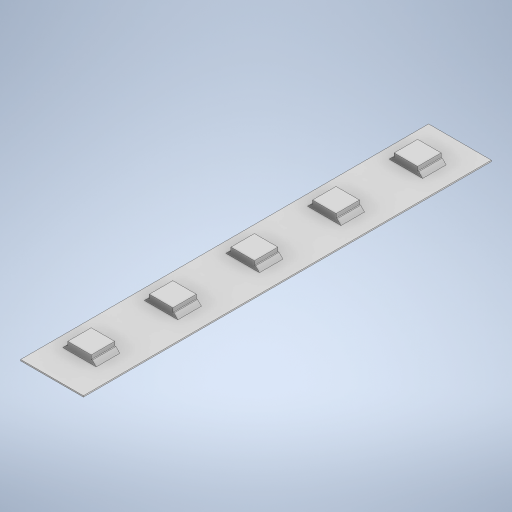
# Autodesk Inventor part: LED_Strip
Saved by Autodesk Inventor 2023 (Build 270158000, 158)
## iProperties
Created: 2022-12-07
Part Number: LED_Strip
Material: Generic
Document SubType Name: Modeling
Designer: spfow
Density: 1 g/cm^3
Appearance: Default
Author: spfow
Autodesk Inventor part; units mm, degrees
ref_plane "YZ Plane" through (0, 0, 0) normal (1, 0, 0) x (0, 1, 0)
ref_plane "XZ Plane" through (0, 0, 0) normal (0, 1, 0) x (-1, 0, 0)
ref_plane "XY Plane" through (0, 0, 0) normal (0, 0, 1) x (1, 0, 0)
sketch "Sketch1" plane through (0, 0, 0) normal (0, 1, 0) x (-1, 0, 0)
  line L0 (0, 0) -> (12.7, 0)
  line L1 (12.7, 0) -> (12.7, 82.55)
  line L2 (12.7, 82.55) -> (0, 82.55)
  line L3 (0, 82.55) -> (0, 0)
  dimension "d0" = 12.7
  dimension "d1" = 82.55
  constraints: 8 end point, 2 parallel, 1 horizontal, 1 perpendicular
  measures "d0" distance of L2.end L1.end
  measures "d1" distance of L0.end L1.end
extrude "Extrusion1" add sketch "Sketch1" along normal blind 0.254
sketch "Sketch2" plane through (0, 0.254, 0) normal (0, 1, 0) x (1, 0, 0)
  line L0 (-9.525, -76.2) -> (-4.7625, -76.2)
  line L1 (-4.7625, -76.2) -> (-4.7625, -71.4375)
  line L2 (-4.7625, -71.4375) -> (-9.525, -71.4375)
  line L3 (-9.525, -71.4375) -> (-9.525, -76.2)
  line L4 (-12.7, -82.55) -> (0, -82.55) projected
  line L5 (-12.7, 0) -> (-12.7, -82.55) projected
  line L6 (-9.525, -59.69) -> (-4.7625, -59.69)
  line L7 (-4.7625, -59.69) -> (-4.7625, -54.9275)
  line L8 (-4.7625, -54.9275) -> (-9.525, -54.9275)
  line L9 (-9.525, -54.9275) -> (-9.525, -59.69)
  line L10 (-9.525, -43.18) -> (-4.7625, -43.18)
  line L11 (-4.7625, -43.18) -> (-4.7625, -38.4175)
  line L12 (-4.7625, -38.4175) -> (-9.525, -38.4175)
  line L13 (-9.525, -38.4175) -> (-9.525, -43.18)
  line L14 (-9.525, -26.67) -> (-4.7625, -26.67)
  line L15 (-4.7625, -26.67) -> (-4.7625, -21.9075)
  line L16 (-4.7625, -21.9075) -> (-9.525, -21.9075)
  line L17 (-9.525, -21.9075) -> (-9.525, -26.67)
  line L18 (-9.525, -10.16) -> (-4.7625, -10.16)
  line L19 (-4.7625, -10.16) -> (-4.7625, -5.3975)
  line L20 (-4.7625, -5.3975) -> (-9.525, -5.3975)
  line L21 (-9.525, -5.3975) -> (-9.525, -10.16)
  line L22 (-4.7625, -59.69) -> (-3.7465, -59.69)
  line L23 (-3.7465, -59.69) -> (-3.7465, -54.9275)
  line L24 (-3.7465, -54.9275) -> (-4.7625, -54.9275)
  line L25 (-4.7625, -54.9275) -> (-4.7625, -59.69)
  line L26 (-4.7625, -76.2) -> (-3.7465, -76.2)
  line L27 (-3.7465, -76.2) -> (-3.7465, -71.4375)
  line L28 (-3.7465, -71.4375) -> (-4.7625, -71.4375)
  line L29 (-4.7625, -71.4375) -> (-4.7625, -76.2)
  line L30 (-9.525, -76.2) -> (-10.541, -76.2)
  line L31 (-10.541, -76.2) -> (-10.541, -71.4375)
  line L32 (-10.541, -71.4375) -> (-9.525, -71.4375)
  line L33 (-9.525, -71.4375) -> (-9.525, -76.2)
  line L34 (-9.525, -59.69) -> (-10.541, -59.69)
  line L35 (-10.541, -59.69) -> (-10.541, -54.9275)
  line L36 (-10.541, -54.9275) -> (-9.525, -54.9275)
  line L37 (-9.525, -54.9275) -> (-9.525, -59.69)
  line L38 (-9.525, -43.18) -> (-10.541, -43.18)
  line L39 (-10.541, -43.18) -> (-10.541, -38.4175)
  line L40 (-10.541, -38.4175) -> (-9.525, -38.4175)
  line L41 (-9.525, -38.4175) -> (-9.525, -43.18)
  line L42 (-4.7625, -43.18) -> (-3.7465, -43.18)
  line L43 (-3.7465, -43.18) -> (-3.7465, -38.4175)
  line L44 (-3.7465, -38.4175) -> (-4.7625, -38.4175)
  line L45 (-4.7625, -38.4175) -> (-4.7625, -43.18)
  line L46 (-4.7625, -26.67) -> (-3.7465, -26.67)
  line L47 (-3.7465, -26.67) -> (-3.7465, -21.9075)
  line L48 (-3.7465, -21.9075) -> (-4.7625, -21.9075)
  line L49 (-4.7625, -21.9075) -> (-4.7625, -26.67)
  line L50 (-9.525, -26.67) -> (-10.541, -26.67)
  line L51 (-10.541, -26.67) -> (-10.541, -21.9075)
  line L52 (-10.541, -21.9075) -> (-9.525, -21.9075)
  line L53 (-9.525, -21.9075) -> (-9.525, -26.67)
  line L54 (-9.525, -10.16) -> (-10.541, -10.16)
  line L55 (-10.541, -10.16) -> (-10.541, -5.3975)
  line L56 (-10.541, -5.3975) -> (-9.525, -5.3975)
  line L57 (-9.525, -5.3975) -> (-9.525, -10.16)
  line L58 (-4.7625, -10.16) -> (-3.7465, -10.16)
  line L59 (-3.7465, -10.16) -> (-3.7465, -5.3975)
  line L60 (-3.7465, -5.3975) -> (-4.7625, -5.3975)
  line L61 (-4.7625, -5.3975) -> (-4.7625, -10.16)
  point P0 (0, 0)
  point P1 (-4.7625, -21.9075)
  point P2 (-4.7625, -54.9275)
  dimension "d4" = 4.7625
  dimension "d5" = 4.7625
  dimension "d6" = 6.35
  dimension "d7" = 3.175
  dimension "d8" = 4.7625
  dimension "d9" = 4.7625
  dimension "d10" = 11.7475
  dimension "d11" = 3.175
  dimension "d12" = 4.7625
  dimension "d13" = 4.7625
  dimension "d14" = 4.7625
  dimension "d15" = 4.7625
  dimension "d16" = 4.7625
  dimension "d17" = 4.7625
  dimension "d18" = 11.7475
  dimension "d19" = 11.7475
  dimension "d20" = 11.7475
  dimension "d21" = 3.175
  dimension "d22" = 1.016
  dimension "d23" = 1.016
  dimension "d31" = 4.7625
  dimension "d32" = 4.7625
  dimension "d33" = 4.7625
  dimension "d34" = 4.7625
  constraints: 120 end point, 30 parallel, 17 point on line, 15 horizontal, 15 perpendicular
  measures "d4" distance of L2.end L0.start
  measures "d5" distance of L0.start L0.end
  measures "d6" distance between parallel lines of L4 L0
  measures "d7" distance between parallel lines of L5 L3
  measures "d8" distance of L8.end L6.start
  measures "d9" distance of L7.end L8.end
  measures "d10" distance between parallel lines of L6 L2
  measures "d11" distance between parallel lines of L5 L9
  measures "d12" distance of L11.end L12.end
  measures "d13" distance of L12.end L10.start
  measures "d14" distance of L16.end L14.start
  measures "d15" distance of L20.end L18.start
  measures "d16" distance of L19.end L20.end
  measures "d17" distance of L15.end L16.end
  measures "d18" distance between parallel lines of L8 L10
  measures "d19" distance between parallel lines of L14 L12
  measures "d20" distance between parallel lines of L18 L16
  measures "d21" distance between parallel lines of L5 L13
  measures "d22" distance of L24.end L23.end
  measures "d23" distance of L31.end L32.end
  measures "d31" distance of L34.end L35.end
  measures "d32" distance of L38.end L39.end
  measures "d33" distance of L50.end L51.end
  measures "d34" distance of L54.end L55.end
extrude "Extrusion2" add sketch "Sketch2" along normal blind 1.5875 contours L3 L2 L1 L0 | L9 L8 L7 L6 | L13 L12 L11 L10 | L17 L16 L15 L14 | L21 L20 L19 L18
extrude "Extrusion3" add sketch "Sketch2" along normal blind 0.7937 contours L30 L31 L32 L3 | L1 L28 L27 L26 | L34 L35 L36 L9 | L7 L24 L23 L22 | L38 L39 L40 L13 | L11 L44 L43 L42 | L50 L51 L52 L17 | L15 L48 L47 L46 | L54 L55 L56 L21 | L19 L60 L59 L58
chamfer "Chamfer1" distance 0.7937 angle 45 10 edges at (-3.7465, 1.0477, 73.8188) (-3.7465, 1.0477, 57.3088) (-3.7465, 1.0477, 40.7988) (-3.7465, 1.0477, 24.2888) (-3.7465, 1.0477, 7.7787) (-10.541, 1.0477, 7.7787) (-10.541, 1.0477, 24.2888) (-10.541, 1.0477, 40.7988) (-10.541, 1.0477, 57.3088) (-10.541, 1.0477, 73.8188)
body "Solid1"
